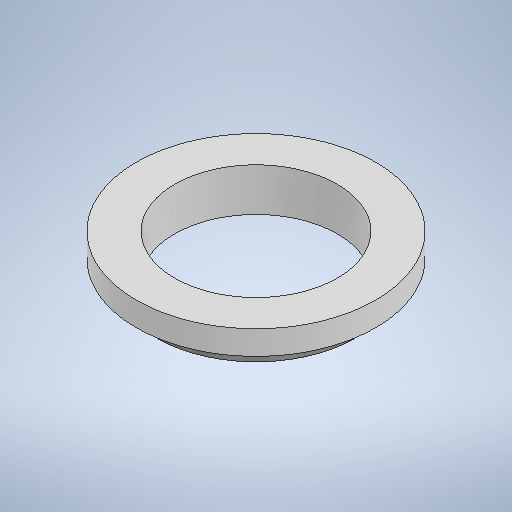
# Autodesk Inventor part: Antriebszahnrad
Saved by Autodesk Inventor 2025 (Build 290162010, 162A)
## iProperties
Created: 2024-11-27
Part Number: Antriebszahnrad
Material: Generisch
Document SubType Name: Modeling
Designer: Jens
Density: 1 g/cm^3
Appearance: Vorgabe
Author: Jens
Autodesk Inventor part; units mm, degrees
ref_plane "YZ Plane" through (0, 0, 0) normal (1, 0, 0) x (0, 1, 0)
ref_plane "XZ Plane" through (0, 0, 0) normal (0, 1, 0) x (-1, 0, 0)
ref_plane "XY Plane" through (0, 0, 0) normal (0, 0, 1) x (1, 0, 0)
sketch "Skizze1" plane through (0, 0, 0) normal (0, 0, 1) x (1, 0, 0)
  circle A0 centre (0, 0) radius 27.5
  circle A1 centre (0, 0) radius 41.5
  circle A2 centre (0, 0) radius 34
  dimension "d0" = 55
  dimension "d1" = 83
  dimension "d2" = 68
  constraints: 3 centre point, 3 coincident
  measures "d0" diameter of A0
  measures "d1" diameter of A1
  measures "d2" diameter of A2
extrude "Extrusion1" add sketch "Skizze1" along normal blind 8 contours A1
sketch "Skizze2" plane through (0, 0, 8) normal (0, 0, 1) x (1, 0, 0)
  circle A0 centre (0, 0) radius 50
  circle A1 centre (0, 0) radius 34
  circle A2 centre (0, 0) radius 34 projected
  dimension "d5" = 100
  constraints: 2 centre point, 2 coincident, 1 concentric
  measures "d5" diameter of A0
extrude "Extrusion2" add sketch "Skizze2" along normal blind 10
